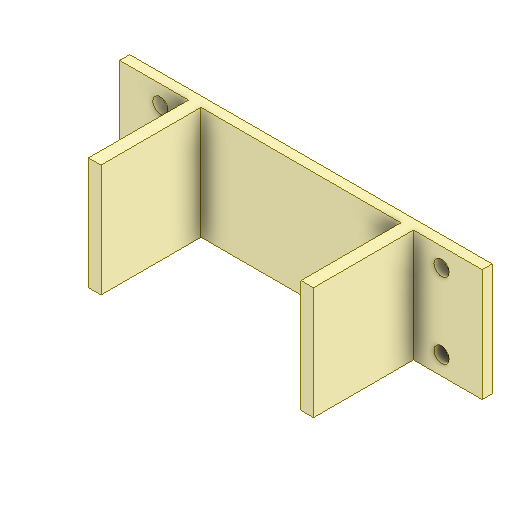
# Autodesk Inventor part: WheelModuleBracket
Saved by Autodesk Inventor 2022 (Build 260153000, 153)
## iProperties
Created: 2024-07-11
Part Number: WheelModuleBracket
Material: ABS Plastic
Document SubType Name: Modeling
Designer: LaptopJR
Density: 1.06 g/cm^3
Appearance: Nylon 6
Author: LaptopJR
Autodesk Inventor part; units mm, degrees
ref_plane "YZ Plane" through (0, 0, 0) normal (1, 0, 0) x (0, 1, 0)
ref_plane "XZ Plane" through (0, 0, 0) normal (0, 1, 0) x (-1, 0, 0)
ref_plane "XY Plane" through (0, 0, 0) normal (0, 0, 1) x (1, 0, 0)
sketch "Sketch1" plane through (0, 0, 0) normal (0, 0, 1) x (1, 0, 0)
  line L0 (-56.25, -15) -> (56.25, -15) construction
  line L1 (56.25, -15) -> (56.25, 15) construction
  line L2 (56.25, 15) -> (-56.25, 15) construction
  line L3 (-56.25, 15) -> (-56.25, -15) construction
  line L4 (-56.25, -15) -> (56.25, 15) construction
  line L5 (56.25, -15) -> (-56.25, 15) construction
  circle A0 centre (-56.25, 15) radius 3.05
  circle A1 centre (56.25, 15) radius 3.05
  circle A2 centre (56.25, -15) radius 3.05
  circle A3 centre (-56.25, -15) radius 3.05
  line L6 (-72.5, -22.5) -> (72.5, -22.5)
  line L7 (72.5, -22.5) -> (72.5, 22.5)
  line L8 (72.5, 22.5) -> (-72.5, 22.5)
  line L9 (-72.5, 22.5) -> (-72.5, -22.5)
  line L10 (-72.5, -22.5) -> (72.5, 22.5) construction
  line L11 (72.5, -22.5) -> (-72.5, 22.5) construction
  point P0 (0, 0)
  dimension "d0" = 112.5
  dimension "d1" = 30
  dimension "d2" = 6.1
  dimension "d3" = 145
  dimension "d4" = 45
  constraints: 24 end point, 4 centre point, 4 coincident, 4 midpoint, 4 parallel, 3 equal radius, 2 horizontal, 2 perpendicular
  measures "d0" distance of L2.end L1.end
  measures "d1" distance of L1.end L0.end
  measures "d2" diameter of A0
  measures "d3" distance of L7.end L8.end
  measures "d4" distance of L8.end L6.start
extrude "Extrusion1" add sketch "Sketch1" along normal blind 4
sketch "Sketch2" plane through (0, 0, 4) normal (0, 0, 1) x (1, 0, 0)
  line L0 (72.5, 22.5) -> (-72.5, 22.5) projected
  line L1 (-72.5, -22.5) -> (72.5, -22.5) projected
  line L2 (-45, 22.5) -> (-40, 22.5)
  line L3 (-40, 22.5) -> (-40, -22.5)
  line L4 (-40, -22.5) -> (-45, -22.5)
  line L5 (-45, -22.5) -> (-45, 22.5)
  line L6 (40, 22.5) -> (45, 22.5)
  line L7 (45, 22.5) -> (45, -22.5)
  line L8 (45, -22.5) -> (40, -22.5)
  line L9 (40, -22.5) -> (40, 22.5)
  line L10 (-72.5, 22.5) -> (-72.5, -22.5) projected
  point P0 (0, 0)
  dimension "d7" = 5
  dimension "d8" = 5
  dimension "d9" = 80
  dimension "d10" = 27.5
  constraints: 16 end point, 4 parallel, 4 point on line, 2 horizontal, 2 perpendicular
  measures "d7" distance between parallel lines of L3 L5
  measures "d8" distance between parallel lines of L7 L9
  measures "d9" distance between parallel lines of L9 L3
  measures "d10" distance between parallel lines of L10 L5
extrude "Extrusion2" add sketch "Sketch2" along normal blind 40 contours L7 L1 L9 L0 | L3 L1 L5 L0
body "Solid1"
